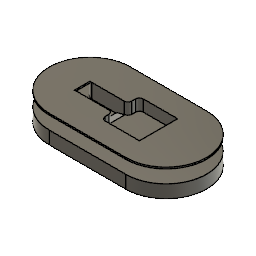
PlayStation Controller Stand v2 (Autodesk Fusion 360 design; units mm, degrees)
Autodesk Fusion 360 part; units mm, degrees
sketch "Sketch1" plane through (0, 0, 0) normal (0, 1, 0) x (1, 0, 0)
  line L0 (0, 0) -> (200, 0)
  line L1 (200, 0) -> (200, -100)
  line L2 (200, -100) -> (0, -100)
  line L3 (0, -100) -> (0, 0)
  line L4 (150, 0) -> (50, 0)
  arc A0 (50, 0) -> (50, -100) centre (50, -50) ccw
  line L5 (50, -100) -> (150, -100)
  arc A1 (150, -100) -> (150, 0) centre (150, -50) ccw
  line L6 (200, -50) -> (0, -50) construction
  arc A2 (150, -77.5) -> (150, -22.5) centre (150, -50) ccw
  line L7 (150, -22.5) -> (50, -22.5)
  arc A3 (50, -22.5) -> (50, -77.5) centre (50, -50) ccw
  line L8 (50, -77.5) -> (150, -77.5)
  arc A4 (150, -110) -> (150, 10) centre (150, -50) ccw
  line L9 (150, 10) -> (50, 10)
  arc A5 (50, 10) -> (50, -110) centre (50, -50) ccw
  line L10 (50, -110) -> (150, -110)
  dimension "d1" = 200
  dimension "d2" = 100
  dimension "d3" = -22.5
  dimension "d47" = 10
  constraint horizontal L0
  constraint vertical L1
  constraint horizontal L2
  constraint vertical L3
  constraint coincident L0.start L3.end
  constraint tangent L4 A0
  constraint tangent A0 L5
  constraint parallel L4 L5
  constraint tangent L5 A1
  constraint tangent L4 A1
  constraint midpoint A1 L6.start
  constraint midpoint A0 L6.end
  constraint midpoint L3 L6.end
  constraint perpendicular L3 L6
  constraint midpoint L1 L6.start
  measures "d1" distance of L0.start L0.end
  measures "d2" distance of L0.start L2.end
extrude "Extrude1" add sketch "Sketch1" along normal blind 19 contours A2 L7 A3 L8 makes body 1
sketch "Sketch2" plane through (0, 19, 0) normal (0, 1, 0) x (-1, 0, 0)
  line L0 (-50, 77.5) -> (-150, 77.5)
  arc A0 (-150, 77.5) -> (-150, 22.5) centre (-150, 50) ccw
  line L1 (-150, 22.5) -> (-50, 22.5)
  arc A1 (-50, 22.5) -> (-50, 77.5) centre (-50, 50) ccw
  line L2 (-150, 22.5) -> (-150, 77.5)
  line L3 (-150, 50) -> (-150, 75)
  line L4 (-150, 75) -> (-100, 75)
  line L5 (-100, 75) -> (-100, 25)
  line L6 (-100, 25) -> (-150, 25)
  line L7 (-150, 25) -> (-150, 75)
  line L8 (-100, 50) -> (-100, 40)
  line L9 (-100, 40) -> (-19.7085, 40)
  line L10 (-19.7085, 40) -> (-19.7085, 60)
  line L11 (-19.7085, 60) -> (-100, 60)
  line L12 (-100, 60) -> (-100, 40)
  dimension "d6" = 25
  dimension "d7" = 50
  dimension "d8" = 50
  dimension "d9" = 10
  dimension "d10" = 20
  constraint coincident A0.end L1.start
  constraint coincident L0.end A0.start
  constraint coincident A0.centre L3.start
  constraint perpendicular L0 L3
  constraint horizontal L4
  constraint vertical L5
  constraint horizontal L6
  constraint vertical L7
  constraint midpoint L5 L8.start
  constraint parallel L5 L8
  constraint horizontal L9
  constraint vertical L10
  constraint horizontal L11
  constraint vertical L12
  measures "d6" distance of A0.centre L3.end
  measures "d7" distance of L3.end L4.end
  measures "d8" distance of L3.end L6.end
  measures "d9" distance of L8.start L8.end
  measures "d10" distance of L8.end L11.end
extrude "Extrude2" cut sketch "Sketch2" against normal blind 19 contours A1 L5 L8 L9 L11 L12 | L2 L3 L4 L5 L6 L7 L8 L12 bodies 1
sketch "Sketch3" plane through (150, 0, 0) normal (-1, 0, 0) x (0, 0, 1)
  line L0 (75, 19) -> (25, 19)
  line L1 (25, 19) -> (25, 0)
  line L2 (25, 0) -> (75, 0)
  line L3 (75, 0) -> (75, 19)
  line L4 (25, 19) -> (75, 19)
  line L5 (75, 19) -> (75, 0)
  line L6 (75, 0) -> (25, 0)
  line L7 (25, 0) -> (25, 19)
  line L8 (25, 9.5) -> (25, 5.75)
  line L9 (25, 5.75) -> (75, 5.75)
  line L10 (75, 5.75) -> (75, 13.25)
  line L11 (75, 13.25) -> (25, 13.25)
  line L12 (25, 13.25) -> (25, 5.75)
  line L13 (50, 13.25) -> (30.2, 13.25)
  line L14 (30.2, 13.25) -> (69.8, 13.25)
  line L15 (69.8, 13.25) -> (69.8, 5.75)
  line L16 (69.8, 5.75) -> (30.2, 5.75)
  line L17 (30.2, 5.75) -> (30.2, 13.25)
  line L18 (50, 5.75) -> (50, 13.25)
  line L19 (50, 9.5) -> (50, 11.65)
  line L20 (50, 11.65) -> (55.65, 11.65)
  line L21 (55.65, 11.65) -> (44.35, 11.65)
  line L22 (44.35, 11.65) -> (44.35, 7.35)
  line L23 (44.35, 7.35) -> (55.65, 7.35)
  line L24 (55.65, 7.35) -> (55.65, 11.65)
  line L25 (44.35, 11.65) -> (43.75, 11.65)
  line L26 (43.75, 11.65) -> (43.75, 7.35)
  line L27 (43.75, 7.35) -> (44.35, 7.35)
  line L28 (44.35, 7.35) -> (44.35, 11.65)
  line L29 (43.75, 11.65) -> (31.95, 11.65)
  line L30 (31.95, 11.65) -> (31.95, 7.35)
  line L31 (31.95, 7.35) -> (43.75, 7.35)
  line L32 (43.75, 7.35) -> (43.75, 11.65)
  line L33 (55.65, 11.65) -> (56.25, 11.65)
  line L34 (56.25, 11.65) -> (56.25, 7.35)
  line L35 (56.25, 7.35) -> (55.65, 7.35)
  line L36 (55.65, 7.35) -> (55.65, 11.65)
  line L37 (56.25, 11.65) -> (68.05, 11.65)
  line L38 (68.05, 11.65) -> (68.05, 7.35)
  line L39 (68.05, 7.35) -> (56.25, 7.35)
  line L40 (56.25, 7.35) -> (56.25, 11.65)
  line L41 (25, 13.25) -> (75, 13.25)
  line L42 (75, 13.25) -> (75, 15.25)
  line L43 (75, 15.25) -> (25, 15.25)
  line L44 (25, 15.25) -> (25, 13.25)
  line L45 (75, 5.75) -> (25, 5.75)
  line L46 (25, 5.75) -> (25, 3.75)
  line L47 (25, 3.75) -> (75, 3.75)
  line L48 (75, 3.75) -> (75, 5.75)
  line L49 (30.2, 3.75) -> (30.2, 15.25)
  line L50 (69.8, 3.75) -> (69.8, 15.25)
  line L51 (69.8, 15.25) -> (71.8, 15.25)
  line L52 (71.8, 15.25) -> (71.8, 3.75)
  line L53 (71.8, 3.75) -> (69.8, 3.75)
  line L54 (69.8, 3.75) -> (69.8, 15.25)
  line L55 (30.2, 15.25) -> (28.2, 15.25)
  line L56 (28.2, 15.25) -> (28.2, 3.75)
  line L57 (28.2, 3.75) -> (30.2, 3.75)
  line L58 (30.2, 3.75) -> (30.2, 15.25)
  dimension "d13" = 3.75
  dimension "d14" = 7.5
  dimension "d15" = 19.8
  dimension "d16" = 39.6
  dimension "d17" = 2.15
  dimension "d18" = 5.65
  dimension "d19" = 11.3
  dimension "d20" = 4.3
  dimension "d21" = 0.6
  dimension "d22" = 11.8
  dimension "d23" = 0.6
  dimension "d24" = 4.3
  dimension "d25" = 11.8
  dimension "d26" = 4.3
  dimension "d28" = 50
  dimension "d29" = 2
  dimension "d30" = 2
  dimension "d31" = 2
  dimension "d32" = 2
  constraint horizontal L4
  constraint vertical L5
  constraint horizontal L6
  constraint vertical L7
  constraint coincident L2.end L3.start
  constraint coincident L0.end L1.start
  constraint midpoint L1 L8.start
  constraint parallel L7 L8
  constraint horizontal L9
  constraint vertical L10
  constraint horizontal L11
  constraint vertical L12
  constraint midpoint L11 L13.start
  constraint parallel L11 L13
  constraint horizontal L14
  constraint vertical L15
  constraint horizontal L16
  constraint vertical L17
  constraint midpoint L16 L18.start
  constraint midpoint L18 L19.start
  constraint perpendicular L14 L19
  constraint perpendicular L19 L20
  constraint horizontal L21
  constraint vertical L22
  constraint horizontal L23
  constraint vertical L24
  constraint horizontal L25
  constraint vertical L26
  constraint horizontal L27
  constraint vertical L28
  constraint horizontal L29
  constraint vertical L30
  constraint horizontal L31
  constraint vertical L32
  constraint horizontal L33
  constraint vertical L34
  constraint horizontal L35
  constraint vertical L36
  constraint horizontal L37
  constraint vertical L38
  constraint horizontal L39
  constraint vertical L40
  constraint horizontal L41
  constraint vertical L42
  constraint horizontal L43
  constraint vertical L44
  constraint horizontal L45
  constraint vertical L46
  constraint horizontal L47
  constraint vertical L48
  constraint coincident L47 L49.start
  constraint coincident L43 L49.end
  constraint perpendicular L43 L49
  constraint coincident L47 L50.start
  constraint coincident L43 L50.end
  constraint perpendicular L43 L50
  constraint horizontal L51
  constraint vertical L52
  constraint horizontal L53
  constraint vertical L54
  constraint horizontal L55
  constraint vertical L56
  constraint horizontal L57
  constraint vertical L58
  measures "d13" distance of L8.start L8.end
  measures "d14" distance of L8.end L11.end
  measures "d15" distance of L13.start L13.end
  measures "d16" distance of L13.end L14.end
  measures "d17" distance of L19.start L19.end
  measures "d18" distance of L19.end L20.end
  measures "d19" distance of L20.end L21.end
  measures "d20" distance of L20.end L23.end
  measures "d21" distance of L21.end L25.end
  measures "d22" distance of L25.end L29.end
  measures "d23" distance of L20.end L33.end
  measures "d24" distance of L20.end L23.end
  measures "d25" distance of L33.end L37.end
  measures "d26" distance of L33.end L34.end
  measures "d28" distance of L11.end L10.end
  measures "d29" distance of L11.end L43.end
  measures "d30" distance of L9.end L47.end
  measures "d31" distance of L50.end L51.end
  measures "d32" distance of L49.end L55.end
extrude "Extrude3" add sketch "Sketch3" along normal blind 3 contours L11 L41 L43 L50 L51 L52 L54 | L11 L41 L43 L49 L55 L56 L58 | L9 L11 L15 L41 L45 L50 L52 L54 | L11 L13 L14 L41 L43 L49 L50 L54 L58 | L9 L11 L17 L41 L45 L49 L56 L58 | L9 L45 L47 L50 L52 L53 L54 | L9 L45 L47 L49 L56 L57 L58 | L9 L16 L45 L47 L49 L50 L54 L58 | L18 L19 L20 L21 L23 L24 L36 | L18 L19 L21 L22 L23 L28 | L34 L37 L38 L39 L40 | L26 L29 L30 L31 L32 bodies 1
extrude "Extrude4" add 1 faces at (150, 1.25, 42.7333) along direction (-1, 0, 0) blind 3 on bodies 1 bodies 1
extrude "Extrude5" add 1 faces at (147, 1.9167, 43.4) along direction (-1, 0, 0) blind 7 on bodies 1 bodies 1
extrude "Extrude6" cut 3 faces at (147, 10.2167, 39.8167) (147, 8.7833, 51.8833) (147, 10.2167, 60.1833) along direction (1, 0, 0) blind 3 on bodies 1 bodies 1
extrude "Extrude7" cut 2 faces at (100, 12.6667, 35) (100, 12.6667, 70) along direction (-1, 0, 0) blind 10 on bodies 1 bodies 1
sketch "Sketch4" plane through (140, 0, 0) normal (-1, 0, 0) x (0, 0, 1)
  line L0 (75, 19) -> (25, 19)
  line L1 (25, 19) -> (25, 0)
  line L2 (25, 0) -> (75, 0)
  line L3 (75, 0) -> (75, 19)
  line L4 (69.8, 13.25) -> (69.8, 5.75)
  line L5 (69.8, 5.75) -> (30.2, 5.75)
  line L6 (30.2, 5.75) -> (30.2, 13.25)
  line L7 (30.2, 13.25) -> (69.8, 13.25)
  line L8 (30.2, 9.5) -> (30.2, 4)
  line L9 (25, 0) -> (75, 0)
  line L10 (75, 0) -> (75, 2)
  line L11 (75, 2) -> (25, 2)
  line L12 (25, 2) -> (25, 0)
  dimension "d43" = 5.5
  dimension "d44" = 2
  constraint midpoint L6 L8.start
  constraint perpendicular L5 L8
  constraint horizontal L9
  constraint vertical L10
  constraint horizontal L11
  constraint vertical L12
  constraint coincident L1.end L2.start
  measures "d43" distance of L8.start L8.end
  measures "d44" distance of L1.end L11.end
extrude "Extrude8" add sketch "Sketch4" along normal blind 50 contours L1 L2 L3 L9 L10 L11 L12 bodies 1
extrude "Extrude9" add sketch "Sketch1" along normal blind 2 contours L0 L2 L4 A0 L5 A1 bodies 1
extrude "Extrude10" add 1 faces at (90, 1.3333, 46.6667) along direction (-1, 0, 0) blind 74 on bodies 1 bodies 1
sketch "Sketch5" plane through (0, 2, 0) normal (0, 1, 0) x (-1, 0, 0)
  arc A0 (-50, 22.5) -> (-24.3826, 40) centre (-50, 50) ccw
  line L0 (-50, 22.5) -> (-150, 22.5)
  arc A1 (-150, 77.5) -> (-150, 22.5) centre (-150, 50) ccw
  line L1 (-150, 77.5) -> (-50, 77.5)
  arc A2 (-24.3826, 60) -> (-50, 77.5) centre (-50, 50) ccw
  line L2 (-24.3826, 60) -> (-90, 60)
  line L3 (-90, 60) -> (-90, 75)
  line L4 (-90, 75) -> (-140, 75)
  line L5 (-140, 75) -> (-140, 25)
  line L6 (-140, 25) -> (-90, 25)
  line L7 (-90, 25) -> (-90, 40)
  line L8 (-90, 40) -> (-24.3826, 40)
  line L9 (-150, 22.5) -> (-75, 22.5)
  line L10 (-75, 22.5) -> (-75, 77.5)
  line L11 (-75, 40) -> (-40, 40)
  line L12 (-40, 40) -> (-40, 60)
  line L13 (-40, 60) -> (-75, 60)
  line L14 (-75, 60) -> (-75, 40)
  arc A3 (-150, 100) -> (-150, 0) centre (-150, 50) ccw
  line L15 (-150, 0) -> (-50, 0)
  arc A4 (-50, 0) -> (-50, 100) centre (-50, 50) ccw
  line L16 (-50, 100) -> (-150, 100)
  dimension "d52" = 75
  dimension "d53" = 35
  constraint coincident L0.end A1.end
  constraint perpendicular L5 L9
  constraint coincident L1 L10.end
  constraint perpendicular L1 L10
  constraint horizontal L11
  constraint vertical L12
  constraint horizontal L13
  constraint vertical L14
  constraint coincident L8 L11.start
  constraint coincident L10 L11.start
  measures "d52" distance of L0.end L9.end
  measures "d53" distance of L11.start L11.end
extrude "Extrude11" cut sketch "Sketch5" against normal blind 2 contours L2 L8 L10 L11 L12 L13 L14 bodies 1
extrude "Extrude12" add 1 faces at (116.6667, 2, 92.5) along direction (0, 1, 0) blind 17 and the other way blind -15 on bodies 1 bodies 1
extrude "Extrude13" cut 1 faces at (116.6667, 2, 92.5) along direction (0, -1, 0) blind 2 on bodies 1 bodies 1
extrude "Extrude14" add sketch "Sketch1" against normal blind 17 separate body contours L0 L2 L4 A0 L5 A1 | A2 L7 A3 L8 makes body 2
fillet "Fillet1" radius 8 2 edges at (24.3826, 8.5, 40) (24.3826, 8.5, 60) on bodies 1
fillet "Fillet2" radius 5 2 edges at (90, 10.5, 60) (90, 10.5, 40) on bodies 1
fillet "Fillet3" radius 5 2 edges at (90, 10.5, 75) (90, 10.5, 25) on bodies 1
extrude "Extrude15" add 1 faces at (123.1827, 2, 54.3076) along direction (0, 1, 0) blind 2 on bodies 1 bodies 1
chamfer "Chamfer1" distance 11 distance2 3 1 edges at (75, 4, 50) measured on face at (123.1827, 4, 54.3076) on bodies 1
move_face "OffsetFaces1" offset 3 1 faces at (83.3333, -5.6667, 0) on bodies 2
move_face "OffsetFaces2" offset 3 1 faces at (83.3333, 18.3333, 0) on bodies 1
equation "d3 = ( -45 / 2 ) * 1 mm"
equation "d70 = 3.75 mm - 1.75 mm"
